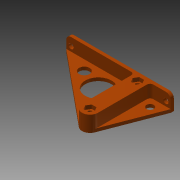
# Autodesk Inventor part: board bracket right
Saved by Autodesk Inventor 2014 (Build 180170000, 170)
## iProperties
Created: 2013-07-23
Part Number: board bracket right
Material: Generic
Document SubType Name: Modeling
Designer: employee
Density: 1 g/cm^3
Mass: 95.7716 g
Surface Area: 299.613 cm^2
Volume: 95.7716 cm^3
Appearance: Smooth - Light Orange
d0: 12.500 mm
d1: 75.000 mm
d2: 8.100 mm
d3: 165.000 mm
d4: 12.500 mm
d5: 5.000 mm
d6: 45.000 mm
d7: 5.000 mm
d8: 0.00 deg
d9: 20.000 mm
d10: 0.00 deg
d11: 8.100 mm
d13: 150.000 mm
d14: 7.500 mm
d15: 12.500 mm
d17: 0.00 deg
d18: 5.000 mm
d19: 13.100 mm
d20: 6.000 mm
d21: 0.00 deg
d31: 7.500 mm
d34: 0.00 deg
d37: 7.500 mm
d40: 0.00 deg
d41: 7.500 mm
d44: 0.00 deg
d45: 7.500 mm
d48: 0.00 deg
d49: 7.500 mm
Author: employee
Autodesk Inventor part; units mm, degrees
ref_plane "YZ Plane" through (0, 0, 0) normal (1, 0, 0) x (0, 1, 0)
ref_plane "XZ Plane" through (0, 0, 0) normal (0, 1, 0) x (-1, 0, 0)
ref_plane "XY Plane" through (0, 0, 0) normal (0, 0, 1) x (1, 0, 0)
sketch "Sketch1" plane through (0, 0, 0) normal (0, 0, 1) x (1, 0, 0)
  line L0 (-120, 0) -> (45, 0)
  circle A0 centre (0, -12.5) radius 4.05
  circle A1 centre (0, -87.5) radius 4.05
  line L1 (-120, 0) -> (-120, -5)
  line L2 (-120, -5) -> (-7.9396, -97.1546)
  arc A2 (-7.9396, -97.1546) -> (11.6724, -91.9728) centre (0, -87.5) ccw
  line L3 (11.6724, -91.9728) -> (45, -5)
  line L4 (45, -5) -> (45, 0)
  point P0 (0, 0)
  dimension "d0" = 12.5
  dimension "d1" = 75
  dimension "d2" = 8.1
  dimension "d3" = 165
  dimension "d4" = 12.5
  dimension "d5" = 5
  dimension "d6" = 45
  constraints: 10 end point, 3 centre point, 2 parallel, 2 point on circle, 2 tangent, 2 vertical alignment, 1 concentric, 1 equal radius, 1 horizontal, 1 perpendicular, 1 point on line
  measures "d0" distance of point (0, 0) A0.centre
  measures "d1" distance of A0.centre A1.centre
  measures "d2" diameter of A0
  measures "d3" distance of L0.start L0.end
  measures "d4" radius of A2
  measures "d5" distance of L0.start L1.end
  measures "d6" horizontal distance of L3.end A0.centre
extrude "Extrusion1" add sketch "Sketch1" along normal blind 5
sketch "Sketch2" plane through (0, 0, 5) normal (0, 0, 1) x (1, 0, 0)
  circle A0 centre (0, -87.5) radius 4.05 projected
  circle A1 centre (0, -12.5) radius 4.05 projected
  line L0 (45, 0) -> (-120, 0) projected
  line L1 (-120, 0) -> (-120, -5) projected
  arc A2 (-7.9396, -97.1546) -> (11.6724, -91.9728) centre (0, -87.5) ccw projected
  line L2 (45, -5) -> (45, 0) projected
  circle A3 centre (0, -87.5) radius 12.5
  line L3 (-120, -5) -> (-12.5, -5)
  line L4 (-12.5, -5) -> (-12.5, -87.5)
  line L5 (12.5, -87.5) -> (12.5, -5)
  line L6 (12.5, -5) -> (45, -5)
  point P0 (0, 0)
  constraints: 8 end point, 3 perpendicular, 3 point on circle, 2 tangent, 1 centre point, 1 coincident, 1 parallel
extrude "Extrusion2" add sketch "Sketch2" along normal blind 20
sketch "Sketch3" plane through (-120, -5, 5) normal (0, -1, 0) x (1, 0, 0)
  line L0 (107.5, 0) -> (0, 0) projected
  line L1 (0, 20) -> (107.5, 20) projected
  line L2 (0, 0) -> (0, 20) projected
  line L3 (165, 0) -> (132.5, 0) projected
  line L4 (165, 0) -> (165, 20) projected
  line L5 (132.5, 20) -> (165, 20) projected
  line L6 (132.5, 0) -> (132.5, 20) projected
  line L7 (7.5, 7.5) -> (157.5, 7.5)
  circle A0 centre (157.5, 7.5) radius 4.05
  circle A1 centre (7.5, 7.5) radius 4.05
  point P0 (120, -5)
  dimension "d11" = 8.1
  dimension "d13" = 150
  dimension "d14" = 7.5
  dimension "d15" = 12.5
  constraints: 2 centre point, 2 coincident, 2 end point, 1 equal radius, 1 parallel, 1 perpendicular
  measures "d11" diameter of A1
  measures "d13" distance of L7.start L7.end
  measures "d14" distance from line of L7.start L2
  measures "d15" distance between parallel lines of L1 L7
extrude "Extrusion3" cut sketch "Sketch3" against normal through all contours A1 | A0
fillet "Fillet1" radius 5 2 edges at (12.5, -5, 15) (-12.5, -5, 15)
sketch "Sketch4" plane through (0, 0, 25) normal (0, 0, 1) x (1, 0, 0)
  circle A0 centre (0, -12.5) radius 4.05 projected
  circle A1 centre (0, -87.5) radius 4.05 projected
  arc A2 (-12.5, -87.5) -> (12.5, -87.5) centre (0, -87.5) ccw projected
  line L0 (7.5633, -12.5) -> (3.7816, -19.05)
  line L1 (3.7816, -19.05) -> (-3.7816, -19.05)
  line L2 (-3.7816, -19.05) -> (-7.5633, -12.5)
  line L3 (-7.5633, -12.5) -> (-3.7816, -5.95)
  line L4 (-3.7816, -5.95) -> (3.7816, -5.95)
  line L5 (3.7816, -5.95) -> (7.5633, -12.5)
  line L6 (7.5633, -87.5) -> (3.7816, -94.05)
  line L7 (3.7816, -94.05) -> (-3.7816, -94.05)
  line L8 (-3.7816, -94.05) -> (-7.5633, -87.5)
  line L9 (-7.5633, -87.5) -> (-3.7816, -80.95)
  line L10 (-3.7816, -80.95) -> (3.7816, -80.95)
  line L11 (3.7816, -80.95) -> (7.5633, -87.5)
  point P0 (0, 0)
  dimension "d19" = 13.1
  constraints: 24 end point, 2 coincident, 2 horizontal, 1 parallel, 26 other
  measures "d19" distance between parallel lines of L7 L10
extrude "Extrusion4" cut sketch "Sketch4" against normal blind 6
sketch "Sketch7" plane through (0, 0, 5) normal (0, 0, 1) x (1, 0, 0)
  line L0 (-120, -5) -> (-7.9396, -97.1546) projected
  circle A0 centre (-40.8613, -33.3613) radius 28.3613
  line L1 (-120, -5) -> (-17.5, -5) projected
  line L2 (-12.5, -10) -> (-12.5, -87.5) projected
  circle A1 centre (-40.8613, -33.3613) radius 20.8613
  point P0 (0, 0)
  dimension "d31" = 7.5
  constraints: 3 tangent, 2 centre point, 1 coincident
  measures "d31" radial gap between concentric circles of A0 A1
extrude "Extrusion7" cut sketch "Sketch7" against normal through all contours A1
sketch "Sketch8" plane through (0, 0, 5) normal (0, 0, 1) x (1, 0, 0)
  circle A0 centre (-40.8613, -33.3613) radius 20.8613 projected
  line L0 (-120, -5) -> (-7.9396, -97.1546) projected
  circle A1 centre (-75.5091, -20.9444) radius 15.9444
  circle A2 centre (-75.5091, -20.9444) radius 8.4444
  line L1 (-120, -5) -> (-17.5, -5) projected
  point P0 (0, 0)
  dimension "d37" = 7.5
  constraints: 3 tangent, 2 centre point, 1 coincident
  measures "d37" radial gap between concentric circles of A2 A1
extrude "Extrusion8" cut sketch "Sketch8" against normal through all contours A2
sketch "Sketch9" plane through (0, 0, 5) normal (0, 0, 1) x (1, 0, 0)
  circle A0 centre (-40.8613, -33.3613) radius 20.8613 projected
  line L0 (-120, -5) -> (-7.9396, -97.1546) projected
  circle A1 centre (-26.13, -64.5485) radius 13.63
  line L1 (-12.5, -10) -> (-12.5, -87.5) projected
  circle A2 centre (-26.13, -64.5485) radius 6.13
  point P0 (0, 0)
  dimension "d41" = 7.5
  constraints: 3 tangent, 2 centre point, 1 coincident
  measures "d41" radial gap between concentric circles of A1 A2
extrude "Extrusion9" cut sketch "Sketch9" against normal through all contours A2
sketch "Sketch10" plane through (0, 0, 5) normal (0, 0, 1) x (1, 0, 0)
  line L0 (11.6724, -91.9728) -> (45, -5) projected
  circle A0 centre (25.7431, -18.2431) radius 13.2431
  line L1 (17.5, -5) -> (45, -5) projected
  line L2 (12.5, -87.5) -> (12.5, -10) projected
  circle A1 centre (25.7431, -18.2431) radius 5.7431
  point P0 (0, 0)
  dimension "d45" = 7.5
  constraints: 3 tangent, 2 centre point, 1 coincident
  measures "d45" radial gap between concentric circles of A0 A1
extrude "Extrusion10" cut sketch "Sketch10" against normal through all contours A1
fillet "Fillet2" radius 7.5 2 edges at (-120, -2.5, 25) (45, -2.5, 25)
body "Solid1"
